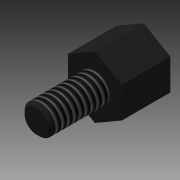
# Autodesk Inventor part: Spacer
Saved by Autodesk Inventor 2015 (Build 190159000, 159)
## iProperties
Created: 2015-10-10
Part Number: Spacer
Material: Nylon 6
Document SubType Name: Modeling
Designer: James
Density: 1.12 g/cm^3
Appearance: Nylon 6
Author: James
Autodesk Inventor part; units mm, degrees
ref_plane "YZ Plane" through (0, 0, 0) normal (1, 0, 0) x (0, 1, 0)
ref_plane "XZ Plane" through (0, 0, 0) normal (0, 1, 0) x (-1, 0, 0)
ref_plane "XY Plane" through (0, 0, 0) normal (0, 0, 1) x (1, 0, 0)
sketch "Sketch1" plane through (0, 0, 0) normal (0, 1, 0) x (-1, 0, 0)
  circle A0 centre (0, 0) radius 1.5
  line L0 (0, 3.1754) -> (2.75, 1.5877)
  line L1 (2.75, 1.5877) -> (2.75, -1.5877)
  line L2 (2.75, -1.5877) -> (0, -3.1754)
  line L3 (0, -3.1754) -> (-2.75, -1.5877)
  line L4 (-2.75, -1.5877) -> (-2.75, 1.5877)
  line L5 (-2.75, 1.5877) -> (0, 3.1754)
  dimension "d0" = 3
  dimension "d4" = 5.5
  constraints: 12 end point, 2 coincident, 1 centre point, 13 other
  measures "d0" diameter of A0
  measures "d4" distance between parallel lines of L1 L4
extrude "Extrusion1" add sketch "Sketch1" along normal blind 5
thread "Thread2" size "M3x0.5" class "6H" standard "ANSI Metric M Profile" full length
sketch "Sketch3" plane through (0, 0, 0) normal (0, -1, 0) x (1, 0, 0)
  circle A0 centre (0, 0) radius 1.5066
  constraints: 1 centre point, 1 coincident
extrude "Extrusion3" add sketch "Sketch3" along normal blind 6
thread "Thread3" size "M3.5x0.6" class "6g" standard "ANSI Metric M Profile" full length
chamfer "Chamfer1" distance 0.3 angle 45 1 edges at (-1.5066, -6, 0)
body "Solid1"
